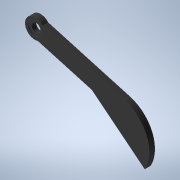
# Autodesk Inventor part: 後ろウィング先端
Saved by Autodesk Inventor 2020.2 (Build 242310000, 310)
## iProperties
Created: 2020-05-05
Part Number: 後ろウィング先端
Material: 一般
Document SubType Name: Modeling
Designer: mozar
Density: 1 g/cm^3
Appearance: 既定
Author: mozar
Autodesk Inventor part; units mm, degrees
ref_plane "YZ Plane" through (0, 0, 0) normal (1, 0, 0) x (0, 1, 0)
ref_plane "XZ Plane" through (0, 0, 0) normal (0, 1, 0) x (-1, 0, 0)
ref_plane "XY Plane" through (0, 0, 0) normal (0, 0, 1) x (1, 0, 0)
sketch "スケッチ1" plane through (0, 0, 0) normal (0, 0, 1) x (1, 0, 0)
  line L0 (-101.5, 47.999998) -> (108.5, 47.999998)
  circle A0 centre (111.885049, -19.000002) radius 4
  circle A1 centre (171.880735, -19.719469) radius 4
  circle A2 centre (111.885049, -19.000002) radius 7
  circle A3 centre (171.880735, -19.719469) radius 7
  line L1 (171.880735, -19.719469) -> (111.885049, -19.000002) construction
  line L2 (171.964673, -12.719973) -> (111.968987, -12.000505)
  line L3 (111.801111, -25.999499) -> (171.796797, -26.718966)
  arc A4 (171.796797, -26.718966) -> (171.964673, -12.719973) centre (171.880735, -19.719469) ccw
  arc A5 (111.968987, -12.000505) -> (111.801111, -25.999499) centre (111.885049, -19.000002) ccw
  line L4 (173.796111, -12.986614) -> (250.19065, -34.719469)
  circle A6 centre (241.981901, -63.574563) radius 30
  line L5 (268.180017, -78.191633) -> (221.951227, -41.241357)
  line L6 (221.951227, -41.241357) -> (169.96536, -26.452325)
  line L7 (271.981901, -113.136134) -> (271.981901, -54.819928)
  line L8 (111.885049, -19.000002) -> (111.885049, 40.999998) construction
  line L9 (118.885049, -19.000002) -> (118.885049, 40.999998)
  line L10 (104.885049, 40.999998) -> (104.885049, -19.000002)
  arc A7 (104.885049, -19.000002) -> (118.885049, -19.000002) centre (111.885049, -19.000002) ccw
  arc A8 (118.885049, 40.999998) -> (104.885049, 40.999998) centre (111.885049, 40.999998) ccw
  circle A9 centre (29.431848, 47.237971) radius 30
  line L11 (113.319325, 34.148513) -> (35.578744, 17.874462)
  line L12 (-0.558472, 47.999998) -> (57.548937, 36.777124)
  line L13 (57.548937, 36.777124) -> (110.450773, 47.851484)
  circle A10 centre (113.5, -20.000002) radius 68
  line L14 (321.963533, -82.955067) -> (60.270532, 100.284345)
  line L15 (259.189194, -39.000002) -> (111.885049, -19.000002)
  arc A11 (93.592427, -27.104845) -> (135.370976, -5.924402) centre (95.060351, 21.794105) ccw
  arc A12 (135.370976, -5.924402) -> (135.847591, -3.671647) centre (132.898992, -4.224609) ccw
  arc A13 (135.847591, -3.671647) -> (83.183341, 18.55647) centre (102.157897, -9.989602) ccw
  line L16 (111.885049, -19.000002) -> (112.689188, 40.994609) construction
  line L17 (118.88442, -19.093818) -> (119.688559, 40.900793)
  line L18 (105.689816, 41.088425) -> (104.885678, -18.906186)
  arc A14 (104.885678, -18.906186) -> (118.88442, -19.093818) centre (111.885049, -19.000002) ccw
  arc A15 (119.688559, 40.900793) -> (105.689816, 41.088425) centre (112.689188, 40.994609) ccw
  line L19 (164.994898, 47.999998) -> (164.994898, 25.999998)
  line L20 (164.994898, 25.999998) -> (327.494898, -102.000002)
  circle A16 centre (116.292557, -40.000002) radius 68
  circle A17 centre (-98.885049, -0.000002) radius 67.5
  line L21 (321.363327, -8.500986) -> (-152.668056, 78.49822)
  line L22 (104.889695, -3) -> (104.889695, 0)
  line L23 (104.889695, -3) -> (72.06562, -3)
  line L24 (72.06562, 0) -> (104.889695, 0)
  circle A18 centre (83.376901, -17.5) radius 13.85
  line L25 (178.77046, -28.957215) -> (174.212284, -32.858886)
  line L26 (174.212284, -32.858886) -> (164.880735, -30.20423)
  line L27 (164.880735, -30.20423) -> (164.880735, -19.719469)
  line L28 (169.96536, -26.452325) -> (168.597236, -31.261507)
  line L29 (168.597236, -31.261507) -> (164.880735, -26.636029)
  line L30 (178.880232, -19.803408) -> (178.654717, -38.608867)
  line L31 (165.012544, -21.071485) -> (158.172386, 13.676274)
  circle A19 centre (171.880735, -19.719469) radius 7.5
  point P0 (0, 0)
  point P1 (0, 0)
  point P2 (141.882892, -19.359736)
  point P3 (111.885049, 10.999998)
  point P4 (105.885049, -0.000002)
  point P5 (105.885049, -0.000002)
  point P6 (23.732778, -42.728965)
  point P7 (112.287118, 10.997304)
  point P8 (169.272284, -12.687685)
  point P9 (163.348193, -12.616644)
  point P10 (164.492485, -18.429603)
  point P11 (172.555184, -27.189082)
  point P12 (178.847945, -22.495796)
  point P13 (170.863298, -26.707772)
  dimension "d0" = 8
  dimension "d1" = 8
  dimension "d2" = 3
  dimension "d3" = 3
  dimension "d4" = 60
  dimension "d5" = 14
  dimension "d6" = 14
  dimension "d7" = 60
  dimension "d8" = 14
  dimension "d9" = 60
  dimension "d10" = 14
  dimension "d11" = 6
  dimension "d12" = 35
  dimension "d13" = 13.271
  dimension "d14" = 14
  dimension "d15" = 20
  dimension "d16" = 15
  dimension "d17" = 22
  dimension "d18" = 150
  dimension "d19" = 162.5
  dimension "d20" = 0
  dimension "d21" = 136
  dimension "d22" = 136
  dimension "d23" = 135
  dimension "d24" = 38.2272
  dimension "d25" = 18
  dimension "d26" = 5
  dimension "d27" = 6
  dimension "d28" = 101.823
  dimension "d29" = 101.823
  dimension "d30" = 0.5
  constraints: 70 end point, 32 point on circle, 30 tangent, 20 centre point, 7 point on line, 5 vertical, 4 equal length, 4 parallel, 3 coincident, 3 horizontal, 3 midpoint, 2 perpendicular, 1 concentric, 10 other
  measures "d0" diameter of A0
  measures "d1" diameter of A1
  measures "d2" radial gap between concentric circles of A0 A2
  measures "d3" radial gap between concentric circles of A1 A3
  measures "d4" distance of L1.start L1.end
  measures "d5" diameter of A5
  measures "d6" distance from line of L4 L5.end
  measures "d7" diameter of A6
  measures "d8" diameter of A8
  measures "d9" diameter of A9
  measures "d10" distance from line of L11 L12.end
  measures "d11" horizontal distance of L1.end point (105.885, 0)
  measures "d12" angle of L14 L0
  measures "d14" diameter of A15
  measures "d15" vertical distance of L15.start L1.end
  measures "d16" vertical distance of L1.start L4.end
  measures "d17" distance of L19.start L19.end
  measures "d18" vertical distance of L19.start L20.end
  measures "d19" distance from line of L19 L20.end
  measures "d20" distance from line of L19.start L0
  measures "d21" diameter of A10
  measures "d22" diameter of A16
  measures "d23" diameter of A17
  measures "d24" angle of L0 L20
  measures "d25" distance from line of L5.start L20
  measures "d26" distance between parallel lines of L6 L26
  measures "d27" distance of L25.start L25.end
  measures "d28" angle of L11 L8
  measures "d29" angle of L1 L31
  measures "d30" radial gap between concentric circles of A3 A19
extrude "押し出し1" add sketch "スケッチ1" against normal blind 5 contours A10 L15 A16 L6 | L6 L30 L15 A10 | A16 L15 A6 L6 | L6 L15 L30 | L15 L30 A19 L4 A16 A10 | A10 A16 L15 | A6 L15 L20 L5 | A16 A10 L4 L20 A6 L15 | L6 A19 L30 L15 | A16 L4 A10 | A6 L20 L15 | L6 L3 A3 L30 A19 | L30 A3 L4 A19 | L20 L4 A6 | A6 L15 L20 | L15 A6 L20 | A3 | A1
hole "穴1" at (105.885049, -0.000002, 0) at (113.5, -20.000002, 0) at (23.732778, -42.728965, 0) at (116.292557, -40.000002, 0) at (-98.885049, -0.000002, 0) at (171.880735, -19.719469, 0) direction (0, 0, -1) diameter 8.05 depth 12 tip angle 118
sketch "スケッチ2" plane through (0, 0, 0) normal (0, 0, 1) x (1, 0, 0)
  circle A0 centre (171.880735, -19.719469) radius 4.025
  arc A1 (268.180017, -78.191633) -> (250.19065, -34.719469) centre (241.981901, -63.574563) ccw
  line L0 (268.180017, -78.191633) -> (221.951227, -41.241357)
  line L1 (221.951227, -41.241357) -> (170.863298, -26.707772)
  line L2 (170.863298, -26.707772) -> (171.796797, -26.718966)
  arc A2 (173.796111, -12.986614) -> (171.796797, -26.718966) centre (171.880735, -19.719469) ccw
  line L3 (173.796111, -12.986614) -> (250.19065, -34.719469)
  circle A3 centre (171.880735, -19.719469) radius 7
  circle A4 centre (171.880735, -19.719469) radius 8.5
  point P0 (0, 0)
  point P1 (178.433917, -14.305986)
  point P2 (174.603168, -27.771696)
  dimension "d40" = 1.5
  constraints: 1 centre point, 1 coincident, 3 other
extrude "押し出し2" add sketch "スケッチ2" against normal blind 5 contours L3 A2 L2 L1 A4
sketch "スケッチ3" plane through (0, 0, 0) normal (0, 0, 1) x (1, 0, 0)
  circle A0 centre (171.880735, -19.719469) radius 4.025
  arc A1 (268.180017, -78.191633) -> (250.19065, -34.719469) centre (241.981901, -63.574563) ccw
  line L0 (268.180017, -78.191633) -> (221.951227, -41.241357)
  line L1 (221.951227, -41.241357) -> (174.603168, -27.771696)
  arc A2 (178.433917, -14.305986) -> (174.603168, -27.771696) centre (171.880735, -19.719469) ccw
  line L2 (178.433917, -14.305986) -> (250.19065, -34.719469)
  circle A3 centre (171.880735, -19.719469) radius 6
  point P0 (0, 0)
  dimension "d43" = 12
  constraints: 1 centre point, 1 coincident
  measures "d43" diameter of A3
extrude "押し出し3" cut sketch "スケッチ3" against normal blind 1 contours A3
equation "\"d9\" = d7"
equation "\"d29\" = d28"
